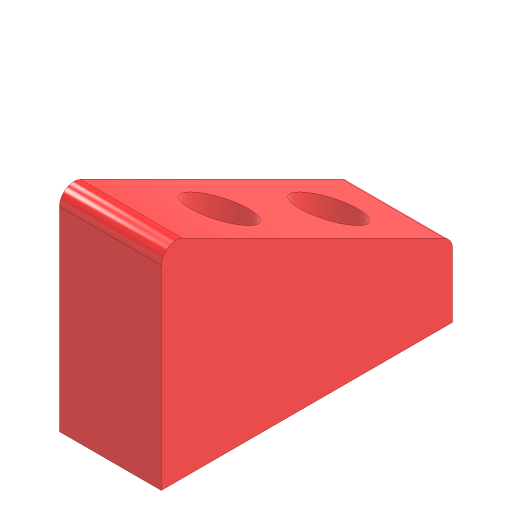
# Autodesk Inventor part: blokada_hiwin
Saved by Autodesk Inventor 2024.3 (Build 283343000, 343)
## iProperties
Created: 2025-06-09
Part Number: blokada_hiwin
Material: Generic
Document SubType Name: Modeling
Designer: MPA
Density: 1 g/cm^3
Appearance: Light Red
Author: MPA
## iProperties of the stored document blokada_hiwin_3DPrint.ipt
Created: 2025-06-18
Part Number: blokada_hiwin_3DPrint
Material: Generic
Document SubType Name: Modeling
Designer: MPA
Density: 1 g/cm^3
Appearance: Default
Author: MPA
Autodesk Inventor part; units mm, degrees
ref_plane "YZ Plane" through (0, 0, 0) normal (1, 0, 0) x (0, 1, 0)
ref_plane "XZ Plane" through (0, 0, 0) normal (0, 1, 0) x (-1, 0, 0)
sketch "Sketch1" plane through (0, 0, 0) normal (1, 0, 0) x (0, 1, 0)
  line L0 (15, 20) -> (-15, 20)
  line L1 (-15, 20) -> (-15, -20)
  line L2 (-15, -20) -> (15, -20)
  line L3 (15, -20) -> (15, 20)
  line L4 (15, 20) -> (-15, -20) construction
  line L5 (-15, 20) -> (15, -20) construction
  point P0 (0, 0)
  dimension "d0" = 30
  dimension "d1" = 40
  constraints: 12 end point, 2 midpoint, 2 parallel, 1 horizontal, 1 perpendicular
  measures "d0" distance of L0.start L0.end
  measures "d1" distance of L2.end L0.start
extrude "Extrusion1" add sketch "Sketch1" along normal blind 14
sketch "Sketch2" plane through (14, 0, 0) normal (1, 0, 0) x (0, 0, -1)
  line L0 (-20, -15) -> (20, -15) projected
  line L1 (20, -15) -> (20, 15) projected
  line L2 (20, 15) -> (-20, 15) projected
  line L3 (-20, 15) -> (-20, -15) projected
  line L4 (-20, 15) -> (20, -5)
  point P0 (0, 0)
  dimension "d4" = 10
  constraints: 2 end point, 1 point on line
  measures "d4" distance of L0.end L4.end
extrude "Extrusion2" cut sketch "Sketch2" against normal through all contours L2 L1 L4
fillet "Fillet1" radius 2 2 edges at (7, 15, 20) (7, -5, -20)
ref_plane "Work Plane1" through (0, -4, -20) normal (0, -1, 0) x (1, 0, 0)
sketch "Sketch3" plane through (0, -4, -20) normal (0, -1, 0) x (1, 0, 0)
  line L0 (0, 40) -> (14, 40) projected
  line L1 (0, 40) -> (14, 40) projected
  line L2 (14, 0) -> (0, 0) projected
  line L3 (0, 0) -> (14, 0) projected
  point P0 (0, 20)
  point P1 (7, 10)
  point P2 (7, 25)
  point P3 (7, 40)
  dimension "d9" = 15
  dimension "d10" = 10
  constraints: 2 vertical alignment, 1 midpoint
  measures "d9" distance of point (7, 10) point (7, 25)
  measures "d10" distance from line of point (7, 10) L2
hole "Hole1" at (7, -4, -10) at (7, -4, 5) direction (0, -1, 0) diameter 4.5 end through all counterbore diameter 8 counterbore depth 4.6 clearance for "Socket Head Cap Screw ISO 4762" size "M4" standard "ISO"
sketch "Sketch4" plane through (0, -4, -20) normal (0, -1, 0) x (1, 0, 0)
  circle A0 centre (7, 10) radius 4 projected
  circle A1 centre (7, 10) radius 4 projected
  circle A2 centre (7, 25) radius 4 projected
  circle A3 centre (7, 25) radius 4 projected
  point P0 (0, 20)
extrude "Extrusion3" cut sketch "Sketch4" against normal through all
body "Solid1"
